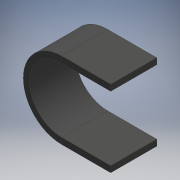
# Autodesk Inventor part: bukket del
Saved by Autodesk Inventor 2018 (Build 220112000, 112)
## iProperties
Created: 2020-08-13
Part Number: bukket del
Material: Steel
Document SubType Name: Sheet Metal
Designer: loppen
Density: 7.85 g/cm^3
Sheet Metal Rule: Default_mm
Appearance: Generic
Flat Pattern Width: 3 cm
Flat Pattern Length: 13.5503 cm
Flat Pattern Area: 40.6508 cm^2
Sheet Metal Width: 30,000 mm
Sheet Metal Length: 135,503 mm
Sheet Metal Area: 4065,079 mm^2
Author: loppen
Autodesk Inventor part; units mm, degrees
ref_plane "YZ Plane" through (0, 0, 0) normal (1, 0, 0) x (0, 1, 0)
ref_plane "XZ Plane" through (0, 0, 0) normal (0, 1, 0) x (-1, 0, 0)
ref_plane "XY Plane" through (0, 0, 0) normal (0, 0, 1) x (1, 0, 0)
sketch "Sketch1" plane through (0, 0, 0) normal (0, 1, 0) x (-1, 0, 0)
  line L0 (0, 0) -> (32, 0)
  arc A0 (32, -50) -> (32, 0) centre (32, -25) ccw
  line L1 (32, -50) -> (0, -50)
  dimension "d11" = 50
  dimension "d12" = 32
  measures "d11" distance between parallel lines of L1 L0
  measures "d12" distance of L0.start L0.end
contour flange "Contour Flange1" sketch "Sketch1" thickness 4 bend radius 4 width 30 along (0, 1, 0) mid plane no both sides no wall seen from (-16, 0, 0) lies toward (0, 0, -1) curves L0 A0 L1
bend "Bend1"
corner "Corner1"
equation "\"d0\" = Thickness"
equation "\"d1\" = BendReliefWidth"
equation "\"d2\" = BendReliefDepth"
equation "\"d3\" = MinimumRemnant"
equation "\"d4\" = TransitionRadius"
equation "\"d6\" = BendRadius"
equation "\"d8\" = CornerReliefSize"
equation "\"d9\" = GapSize"
equation "\"d10\" = JacobiRadiusSize"
equation "\"BendRadius\" = Thickness"
equation "\"BendReliefWidth\" = Thickness"
equation "\"BendReliefDepth\" = 0.5 * Thickness"
equation "\"CornerReliefSize\" = 4 * Thickness"
equation "\"MinimumRemnant\" = 2 * Thickness"
equation "\"TransitionRadius\" = BendRadius"
equation "\"JacobiRadiusSize\" = BendRadius"
equation "\"GapSize\" = Thickness"
equation "\"Thickness\" = 4"
body "Solid1"
